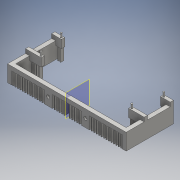
# Autodesk Inventor part: XBOX holder
Saved by Autodesk Inventor 2016 SP2 (Build 200236200, 236)
## iProperties
Created: 2018-02-19
Part Number: XBOX holder
Material: Generic
Document SubType Name: Modeling
Designer: Alexander
Density: 1 g/cm^3
Appearance: Default
Author: Alexander
Autodesk Inventor part; units mm, degrees
ref_plane "YZ Plane" through (0, 0, 0) normal (1, 0, 0) x (0, 1, 0)
ref_plane "XZ Plane" through (0, 0, 0) normal (0, 1, 0) x (-1, 0, 0)
ref_plane "XY Plane" through (0, 0, 0) normal (0, 0, 1) x (1, 0, 0)
sketch "Sketch1" plane through (0, 0, 0) normal (0, 0, 1) x (1, 0, 0)
  line L0 (-57.6, 21) -> (-53.6, 21)
  line L1 (-53.6, 21) -> (-53.6, 17)
  line L2 (-53.6, 17) -> (-57.6, 17)
  line L3 (-57.6, 17) -> (-57.6, 21)
  line L4 (53.6, 21) -> (57.6, 21)
  line L5 (57.6, 21) -> (57.6, 17)
  line L6 (57.6, 17) -> (53.6, 17)
  line L7 (53.6, 17) -> (53.6, 21)
  line L8 (-57.6, 17) -> (-67.6, 17)
  line L9 (-67.6, 17) -> (-67.6, 0)
  line L10 (-67.6, 0) -> (67.6, 0)
  line L11 (67.6, 0) -> (67.6, 17)
  line L12 (67.6, 17) -> (57.6, 17)
  line L13 (-57.6, 21) -> (-53.6, 17) construction
  line L14 (53.6, 17) -> (57.6, 21) construction
  line L15 (-57.6, 21) -> (-72.6, 21)
  line L16 (-72.6, 21) -> (-72.6, -5)
  line L17 (-72.6, -5) -> (72.6, -5)
  line L18 (72.6, -5) -> (72.6, 21)
  line L19 (72.6, 21) -> (57.6, 21)
  point P0 (0, 0)
  point P1 (-55.6, 19)
  point P2 (55.6, 19)
  point P3 (0, 0)
  dimension "d0" = 4
  dimension "d1" = 4
  dimension "d2" = 4
  dimension "d3" = 4
  dimension "d4" = 17
  dimension "d5" = 17
  dimension "d6" = 111.2
  dimension "d7" = 5
  dimension "d8" = 5
  dimension "d9" = 5
  dimension "d10" = 10
  constraints: 40 end point, 7 perpendicular, 5 horizontal, 4 parallel, 3 midpoint, 1 coincident, 1 collinear, 1 point on line, 1 vertical
  measures "d0" distance of L0.start L0.end
  measures "d1" distance of L0.end L1.end
  measures "d2" distance of L4.start L4.end
  measures "d3" distance of L4.end L5.end
  measures "d4" distance of L8.end L9.end
  measures "d5" distance of L10.end L11.end
  measures "d6" distance of point (55.6, 19) point (-55.6, 19)
  measures "d7" distance between parallel lines of L9 L16
  measures "d8" distance between parallel lines of L18 L11
  measures "d9" distance between parallel lines of L17 L10
  measures "d10" distance of L2.end L8.end
extrude "Frame" add sketch "Sketch1" along normal blind 5
sketch "Sketch2" plane through (0, 0, 5) normal (0, 0, 1) x (1, 0, 0)
  line L0 (-67.6, 17) -> (-53.6, 17) projected
  line L1 (-53.6, 17) -> (-57.6, 17)
  line L2 (-57.6, 17) -> (-57.6, 21) construction
  line L3 (-53.6, 21) -> (-72.6, 21) projected
  line L4 (-57.6, 21) -> (-53.6, 17) construction
  circle A0 centre (-55.6, 19) radius 1
  line L5 (0, 0) -> (0, -5.6301) construction
  circle A1 centre (55.6, 19) radius 1
  dimension "d13" = 4
  dimension "d14" = 2
  constraints: 8 end point, 2 centre point, 2 point on line, 1 midpoint, 1 perpendicular, 1 symmetric about line, 1 vertical, 1 other
  measures "d13" distance of L0.end L1.end
  measures "d14" diameter of A0
extrude "Pins" add sketch "Sketch2" along normal blind 10
sketch "Sketch3" plane through (0, 0, 0) normal (0, 0, -1) x (-1, 0, 0)
  line L0 (17.75, -5) -> (-17.75, -5)
  line L1 (72.6, -5) -> (-72.6, -5) projected
  line L2 (72.6, -5) -> (-72.6, -5) projected
  line L3 (17.75, -5) -> (27.75, -5)
  line L4 (27.75, -5) -> (27.75, 0)
  line L5 (27.75, 0) -> (17.75, 0)
  line L6 (17.75, 0) -> (17.75, -5)
  line L7 (0, -5) -> (0, 0) construction
  line L8 (-17.75, -5) -> (-27.75, -5)
  line L9 (-27.75, -5) -> (-27.75, 0)
  line L10 (-27.75, 0) -> (-17.75, 0)
  line L11 (-17.75, 0) -> (-17.75, -5)
  point P0 (0, -5)
  dimension "d17" = 35.5
  dimension "d18" = 10
  dimension "d19" = 5
  constraints: 20 end point, 3 midpoint, 3 symmetric about line, 2 perpendicular, 2 vertical, 1 horizontal, 1 point on line
  measures "d17" distance of L0.start L0.end
  measures "d18" distance of L0.start L3.end
  measures "d19" distance of L3.end L4.end
extrude "Connection Points" add sketch "Sketch3" along normal blind 15
sketch "Sketch4" plane through (-72.6, -5, 5) normal (0, -1, 0) x (1, 0, 0)
  line L0 (44.85, -5) -> (5, -5) projected
  line L1 (44.85, -5) -> (54.85, -5) construction
  line L2 (49.85, -5) -> (49.85, -10) construction
  circle A0 centre (49.85, -10) radius 2
  line L3 (72.6, -5) -> (72.6, 0.0988) construction
  circle A1 centre (95.35, -10) radius 2
  dimension "d22" = 5
  dimension "d23" = 4
  constraints: 6 end point, 2 centre point, 2 vertical, 1 coincident, 1 horizontal, 1 midpoint, 1 symmetric about line, 1 other
  measures "d22" distance of L2.start L2.end
  measures "d23" diameter of A0
extrude "Nail Holes" cut sketch "Sketch4" against normal up to next
sketch "Sketch6" plane through (0, 0, 0) normal (0, 0, -1) x (-1, 0, 0)
  line L0 (-53.6, 17) -> (-67.6, 17) projected
  line L1 (-72.6, 21) -> (-53.6, 21) projected
  line L2 (-67.6, 21) -> (-67.6, 17)
  line L3 (-67.6, 17) -> (-72.6, 17)
  line L4 (-72.6, -5) -> (-72.6, 21) projected
  line L5 (0, 0) -> (0, -5) construction
  line L6 (72.6, -5) -> (-72.6, -5) projected
  line L7 (67.6, 21) -> (67.6, 17)
  line L8 (67.6, 17) -> (72.6, 17)
  line L9 (-72.6, 8) -> (-69.6, 8) construction
  line L10 (-67.6, -5) -> (-67.6, -1)
  line L11 (-67.6, -1) -> (-72.6, -1)
  line L12 (67.6, -1) -> (72.6, -1)
  line L13 (67.6, -5) -> (67.6, -1)
  line L14 (72.6, 21) -> (72.6, -5) projected
  line L15 (53.6, 21) -> (72.6, 21) projected
  line L16 (67.6, -5) -> (72.6, -5)
  line L17 (72.6, -1) -> (72.6, -5)
  line L18 (-72.6, -1) -> (-72.6, -5)
  line L19 (-72.6, -5) -> (-67.6, -5)
  line L20 (67.6, 21) -> (72.6, 21)
  line L21 (72.6, 21) -> (72.6, 17)
  point P0 (72.6, 8)
  point P1 (63.1, 21)
  constraints: 32 end point, 9 symmetric about line, 4 horizontal, 4 midpoint, 3 vertical, 2 point on line, 1 collinear, 1 perpendicular
extrude "Legs" add sketch "Sketch6" along normal blind 15
sketch "Sketch8" plane through (-72.6, 17, 0) normal (0, -1, 0) x (1, 0, 0)
  line L0 (5, 0) -> (5, -15) projected
  line L1 (5, 0) -> (0, 0)
  line L2 (0, -15) -> (0, 5) projected
  line L3 (0, 0) -> (0, -15)
  line L4 (0, -15) -> (5, -15)
  point P0 (72.6, 0)
  constraints: 6 end point, 2 perpendicular, 1 horizontal
extrude "Lower Rim 1" add sketch "Sketch8" along normal up to next
ref_plane "Midplane vertical" through (0, 0, 5) normal (-1, 0, 0) x (0, 0, 1)
mirror "Lower Rim Mirror 1" about plane through (0, 0, 5) normal (-1, 0, 0) of "Lower Rim 1"
sketch "Sketch11" plane through (0, 0, 0) normal (0, 0, -1) x (-1, 0, 0)
  line L0 (-67.6, 21) -> (-53.6, 21)
  line L1 (-53.6, 17) -> (-67.6, 17)
  line L2 (-65.6, 21) -> (-64.6, 21)
  line L3 (-64.6, 21) -> (-64.6, 17)
  line L4 (-64.6, 17) -> (-65.6, 17)
  line L5 (-65.6, 17) -> (-65.6, 21)
  line L6 (-67.6, 17) -> (-67.6, 21)
  line L7 (-62.6, 21) -> (-61.6, 21)
  line L8 (-61.6, 21) -> (-61.6, 17)
  line L9 (-61.6, 17) -> (-62.6, 17)
  line L10 (-62.6, 17) -> (-62.6, 21)
  line L11 (-53.6, 17) -> (-67.6, 17)
  line L12 (-59.6, 21) -> (-58.6, 21)
  line L13 (-58.6, 21) -> (-58.6, 17)
  line L14 (-58.6, 17) -> (-59.6, 17)
  line L15 (-59.6, 17) -> (-59.6, 21)
  line L16 (-56.6, 17) -> (-56.6, 21)
  line L17 (-56.6, 21) -> (-55.6, 21)
  line L18 (-55.6, 17) -> (-56.6, 17)
  line L19 (-55.6, 21) -> (-55.6, 17)
  line L20 (0, 0) -> (0, -5) construction
  line L21 (17.75, -5) -> (-17.75, -5)
  line L22 (53.6, 17) -> (67.6, 17)
  line L23 (53.6, 17) -> (67.6, 17)
  line L24 (67.6, 21) -> (53.6, 21)
  line L25 (59.6, 17) -> (59.6, 21)
  line L26 (59.6, 21) -> (58.6, 21)
  line L27 (58.6, 17) -> (59.6, 17)
  line L28 (58.6, 21) -> (58.6, 17)
  line L29 (56.6, 17) -> (56.6, 21)
  line L30 (55.6, 21) -> (55.6, 17)
  line L31 (55.6, 17) -> (56.6, 17)
  line L32 (56.6, 21) -> (55.6, 21)
  line L33 (65.6, 21) -> (64.6, 21)
  line L34 (64.6, 21) -> (64.6, 17)
  line L35 (62.6, 21) -> (61.6, 21)
  line L36 (61.6, 17) -> (62.6, 17)
  line L37 (61.6, 21) -> (61.6, 17)
  line L38 (64.6, 17) -> (65.6, 17)
  line L39 (65.6, 17) -> (65.6, 21)
  line L40 (67.6, 17) -> (67.6, 21)
  line L41 (62.6, 17) -> (62.6, 21)
  line L42 (-67.6, -5) -> (-67.6, 21) projected
  line L43 (67.6, 21) -> (67.6, -5) projected
  line L44 (64.6, 21) -> (65.6, 21)
  line L45 (65.6, 17) -> (64.6, 17)
  line L46 (67.6, 17) -> (53.6, 17) projected
  point P0 (-62.1, 21)
  point P1 (-62.1, 17)
  point P2 (-59.1, 17)
  point P3 (-59.1, 21)
  point P4 (-56.1, 17)
  point P5 (-56.1, 21)
  point P6 (59.1, 17)
  point P7 (59.1, 21)
  point P8 (56.1, 17)
  point P9 (56.1, 21)
  point P10 (62.1, 21)
  point P11 (62.1, 17)
  point P12 (-67.6, 0)
  point P13 (-67.6, 19)
  point P14 (67.6, 0)
  dimension "d47" = 1
  dimension "d48" = 2
  dimension "d49" = 1
  dimension "d50" = 2
  dimension "d51" = 1
  dimension "d52" = 2
  dimension "d53" = 1
  dimension "d54" = 2
  dimension "d55" = 4
  constraints: 88 end point, 26 symmetric about line, 18 point on line, 8 midpoint, 8 parallel, 4 horizontal, 4 perpendicular, 2 collinear
  measures "d47" distance between parallel lines of L3 L5
  measures "d48" distance between parallel lines of L5 L6
  measures "d49" distance between parallel lines of L8 L10
  measures "d50" distance between parallel lines of L3 L10
  measures "d51" distance between parallel lines of L13 L15
  measures "d52" distance between parallel lines of L15 L8
  measures "d53" distance between parallel lines of L19 L16
  measures "d54" distance between parallel lines of L16 L13
  measures "d55" distance between parallel lines of L1 L0
extrude "Supports Peg" add sketch "Sketch11" along normal blind 15 contours L0 L3 L1 L5 | L0 L8 L1 L10 | L0 L13 L1 L15 | L0 L19 L1 L16 | L30 L24 L29 L22 | L28 L24 L25 L22 | L37 L24 L41 L22 | L34 L24 L39 L22
sketch "Sketch12" plane through (-67.6, 0, 5) normal (0, 1, 0) x (1, 0, 0)
  circle A0 centre (90.35, 10) radius 2 projected
  circle A1 centre (90.35, 10) radius 3
  circle A2 centre (44.85, 10) radius 2 projected
  circle A3 centre (44.85, 10) radius 3
  point P0 (67.6, 5)
  dimension "d58" = 6
  dimension "d59" = 6
  constraints: 2 centre point, 2 coincident
  measures "d58" diameter of A1
  measures "d59" diameter of A3
extrude "Nail Heads" cut sketch "Sketch12" against normal blind 3
sketch "Sketch13" plane through (0, 0, 0) normal (0, 0, -1) x (-1, 0, 0)
  line L0 (27.75, 0) -> (67.6, 0) projected
  line L1 (27.75, 0) -> (29.75, 0)
  line L2 (29.75, 0) -> (29.75, -5)
  line L3 (67.6, -5) -> (27.75, -5) projected
  line L4 (29.75, -5) -> (30.75, -5)
  line L5 (30.75, -5) -> (30.75, 0)
  line L6 (29.75, 0) -> (32.75, 0)
  line L7 (32.75, 0) -> (32.75, -5)
  line L8 (32.75, -5) -> (33.75, -5)
  line L9 (33.75, -5) -> (33.75, 0)
  line L10 (32.75, 0) -> (33.75, 0)
  line L11 (33.75, 0) -> (35.75, 0)
  line L12 (35.75, 0) -> (35.75, -5)
  line L13 (35.75, -5) -> (36.75, -5)
  line L14 (36.75, -5) -> (36.75, 0)
  line L15 (35.75, 0) -> (36.75, 0)
  line L16 (36.75, 0) -> (38.75, 0)
  line L17 (38.75, 0) -> (38.75, -5)
  line L18 (38.75, -5) -> (39.75, -5)
  line L19 (39.75, -5) -> (39.75, 0)
  line L20 (38.75, 0) -> (39.75, 0)
  line L21 (39.75, 0) -> (41.75, 0)
  line L22 (41.75, 0) -> (41.75, -5)
  line L23 (41.75, -5) -> (42.75, -5)
  line L24 (42.75, -5) -> (42.75, 0)
  line L25 (41.75, 0) -> (42.75, 0)
  line L26 (42.75, 0) -> (44.75, 0)
  line L27 (44.75, 0) -> (44.75, -5)
  line L28 (44.75, -5) -> (45.75, -5)
  line L29 (45.75, -5) -> (45.75, 0)
  line L30 (44.75, 0) -> (45.75, 0)
  line L31 (45.75, 0) -> (47.75, 0)
  line L32 (47.75, 0) -> (47.75, -5)
  line L33 (72.6, -5) -> (-72.6, -5) projected
  line L34 (47.75, -5) -> (48.75, -5)
  line L35 (48.75, -5) -> (48.75, 0)
  line L36 (-67.6, 0) -> (67.6, 0) projected
  line L37 (47.8501, 0) -> (48.75, 0)
  line L38 (48.75, 0) -> (50.75, 0)
  line L39 (50.75, 0) -> (50.75, -5)
  line L40 (50.75, -5) -> (51.75, -5)
  line L41 (51.75, -5) -> (51.75, 0)
  line L42 (50.75, 0) -> (51.75, 0)
  line L43 (51.75, 0) -> (50.75, 0)
  line L44 (51.75, 0) -> (53.75, 0)
  line L45 (53.75, 0) -> (53.75, -5)
  line L46 (53.75, -5) -> (54.75, -5)
  line L47 (54.75, -5) -> (54.75, 0)
  line L48 (53.75, 0) -> (54.75, 0)
  line L49 (54.75, 0) -> (56.75, 0)
  line L50 (56.75, 0) -> (56.75, -5)
  line L51 (56.75, -5) -> (57.75, -5)
  line L52 (57.75, -5) -> (57.75, 0)
  line L53 (56.75, 0) -> (57.75, 0)
  line L54 (57.75, 0) -> (59.75, 0)
  line L55 (59.75, 0) -> (59.75, -5)
  line L56 (59.75, -5) -> (60.75, -5)
  line L57 (60.75, -5) -> (60.75, 0)
  line L58 (59.75, 0) -> (60.75, 0)
  line L59 (60.75, 0) -> (62.75, 0)
  line L60 (62.75, 0) -> (62.75, -5)
  line L61 (62.75, -5) -> (63.75, -5)
  line L62 (63.75, -5) -> (63.75, 0)
  line L63 (62.75, 0) -> (63.75, 0)
  line L64 (63.75, 0) -> (65.75, 0)
  line L65 (65.75, 0) -> (65.75, -5)
  line L66 (65.75, -5) -> (66.75, -5)
  line L67 (66.75, -5) -> (66.75, 0)
  line L68 (65.75, 0) -> (66.75, 0)
  line L69 (47.8501, 0) -> (47.75, 0)
  point P0 (0, 0)
  dimension "d62" = 2
  dimension "d63" = 1
  dimension "d64" = 3
  dimension "d65" = 1
  dimension "d66" = 2
  dimension "d67" = 1
  dimension "d68" = 2
  dimension "d69" = 1
  dimension "d70" = 2
  dimension "d71" = 1
  dimension "d72" = 2
  dimension "d73" = 1
  dimension "d74" = 2
  dimension "d75" = 1
  dimension "d76" = 2
  dimension "d77" = 1
  dimension "d78" = 2
  dimension "d79" = 1
  dimension "d80" = 2
  dimension "d81" = 1
  dimension "d82" = 2
  dimension "d83" = 1
  dimension "d84" = 2
  dimension "d85" = 1
  dimension "d86" = 2
  dimension "d87" = 1
  constraints: 132 end point, 25 vertical, 8 perpendicular, 7 horizontal, 57 other
  measures "d62" distance of L1.start L1.end
  measures "d63" distance of L2.end L4.end
  measures "d64" distance of L1.end L6.end
  measures "d65" distance of L7.end L8.end
  measures "d66" distance of L9.end L11.end
  measures "d67" distance of L12.end L13.end
  measures "d68" distance of L14.end L16.end
  measures "d69" distance of L17.end L18.end
  measures "d70" distance of L19.end L21.end
  measures "d71" distance of L22.end L23.end
  measures "d72" distance of L24.end L26.end
  measures "d73" distance of L27.end L28.end
  measures "d74" distance of L29.end L31.end
  measures "d75" distance of L32.end L34.end
  measures "d76" distance of L35.end L38.end
  measures "d77" distance of L39.end L40.end
  measures "d78" distance of L41.end L44.end
  measures "d79" distance of L45.end L46.end
  measures "d80" distance of L47.end L49.end
  measures "d81" distance of L50.end L51.end
  measures "d82" distance of L52.end L54.end
  measures "d83" distance of L55.end L56.end
  measures "d84" distance of L57.end L59.end
  measures "d85" distance of L60.end L61.end
  measures "d86" distance of L62.end L64.end
  measures "d87" distance of L65.end L66.end
extrude "Supports Front" add sketch "Sketch13" along normal blind 15 contours L0 L5 L3 L2 | L0 L9 L3 L7 | L0 L14 L3 L12 | L0 L19 L3 L17 | L0 L24 L3 L22 | L0 L29 L3 L27 | L0 L35 L3 L32 | L0 L41 L3 L39 | L0 L47 L3 L45 | L0 L52 L3 L50 | L0 L57 L3 L55 | L0 L62 L3 L60 | L0 L67 L3 L65
mirror "Mirror3" about plane through (0, 0, 5) normal (-1, 0, 0) of "Supports Front"
sketch "Sketch14" plane through (0, 0, 0) normal (0, 0, -1) x (-1, 0, 0)
  line L0 (17.75, -5) -> (-17.75, -5) construction
  line L1 (17.75, -5) -> (15.75, -5)
  line L2 (15.75, -5) -> (15.75, 0)
  line L3 (15.75, 0) -> (14.75, 0)
  line L4 (-17.75, 0) -> (17.75, 0) construction
  line L5 (14.75, 0) -> (14.75, -5)
  line L6 (15.75, -5) -> (14.75, -5)
  line L7 (14.75, 0) -> (12.75, 0)
  line L8 (12.75, 0) -> (12.75, -5)
  line L9 (12.75, -5) -> (11.75, -5)
  line L10 (11.75, -5) -> (11.75, 0)
  line L11 (12.75, 0) -> (11.75, 0)
  line L12 (11.75, -5) -> (9.75, -5)
  line L13 (9.75, -5) -> (9.75, 0)
  line L14 (9.75, 0) -> (8.75, 0)
  line L15 (8.75, 0) -> (8.75, -5)
  line L16 (9.75, -5) -> (8.75, -5)
  line L17 (8.75, -5) -> (6.75, -5)
  line L18 (6.75, -5) -> (6.75, 0)
  line L19 (6.75, 0) -> (5.75, 0)
  line L20 (5.75, 0) -> (5.75, -5)
  line L21 (6.75, -5) -> (5.75, -5)
  line L22 (5.75, -5) -> (3.75, -5)
  line L23 (3.75, -5) -> (3.75, 0)
  line L24 (3.75, -5) -> (2.75, -5)
  line L25 (72.6, -5) -> (-72.6, -5) projected
  line L26 (2.75, -5) -> (2.75, 0)
  line L27 (3.75, 0) -> (2.75, 0)
  line L28 (2.75, -5) -> (0.75, -5)
  point P0 (0, 0)
  dimension "d90" = 2
  dimension "d91" = 1
  dimension "d92" = 5
  dimension "d93" = 2
  dimension "d94" = 1
  dimension "d95" = 2
  dimension "d96" = 1
  dimension "d97" = 2
  dimension "d98" = 1
  dimension "d99" = 2
  dimension "d100" = 1
  dimension "d101" = 2
  constraints: 52 end point, 6 vertical, 5 horizontal, 4 perpendicular, 2 point on line, 20 other
  measures "d90" distance of L1.start L1.end
  measures "d91" distance of L2.end L3.end
  measures "d92" distance of L1.end L2.end
  measures "d93" distance of L3.end L7.end
  measures "d94" distance of L8.end L9.end
  measures "d95" distance of L9.end L12.end
  measures "d96" distance of L13.end L14.end
  measures "d97" distance of L15.end L17.end
  measures "d98" distance of L18.end L19.end
  measures "d99" distance of L20.end L22.end
  measures "d100" distance of L22.end L24.end
  measures "d101" distance of L24.end L28.end
extrude "Internal Supports Front" add sketch "Sketch14" along normal blind 15 contours L6 L5 L3 L2 | L24 L26 L27 L23 | L21 L20 L19 L18 | L16 L15 L14 L13 | L9 L10 L11 L8
mirror "Mirror4" about plane through (0, 0, 5) normal (-1, 0, 0) of "Internal Supports Front"
sketch "Sketch15" plane through (-72.6, 21, 5) normal (0, 1, 0) x (1, 0, 0)
  line L0 (140.2, 5) -> (140.2, 20) projected
  line L1 (140.2, 5) -> (140.2, 0) projected
  line L2 (140.2, 20) -> (140.2, 0)
  line L3 (140.2, 0) -> (145.2, 0)
  line L4 (145.2, 20) -> (145.2, 0) projected
  line L5 (145.2, 0) -> (145.2, 20)
  line L6 (145.2, 20) -> (140.2, 20)
  line L7 (5, 5) -> (5, 0) projected
  line L8 (5, 0) -> (5, 20)
  line L9 (0, 20) -> (5, 20) projected
  line L10 (5, 20) -> (0, 20)
  line L11 (0, 20) -> (0, 0) projected
  line L12 (0, 20) -> (0, 0)
  line L13 (0, 0) -> (5, 0)
  point P0 (72.6, 5)
  constraints: 16 end point, 6 perpendicular, 2 vertical
extrude "Side Frame Extension" add sketch "Sketch15" along normal blind 40
sketch "Sketch16" plane through (67.6, 0, 5) normal (-1, 0, 0) x (0, 0, 1)
  line L0 (0, 21) -> (0, 61) projected
  line L1 (0, 52.928) -> (-5, 52.928)
  line L2 (-5, 52.928) -> (-5, 48.928)
  line L3 (-5, 48.928) -> (0, 48.928)
  line L4 (0, 48.928) -> (0, 52.928)
  line L5 (-5, 17) -> (0, 17) projected
  line L6 (0, 17) -> (0, 21)
  point P0 (-5, 0)
  point P1 (0, 19)
  point P2 (0, 50.928)
  dimension "d106" = 5
  dimension "d107" = 4
  dimension "d108" = 31.928
  constraints: 10 end point, 2 midpoint, 2 parallel, 1 horizontal, 1 perpendicular, 1 point on line, 1 vertical
  measures "d106" distance of L3.end L2.end
  measures "d107" distance of L1.end L2.end
  measures "d108" distance of point (0, 19) point (0, 50.928)
extrude "Back Bar" add sketch "Sketch16" along normal blind 7
mirror "Between two Rows" about plane through (0, 0, 5) normal (-1, 0, 0) of "Back Bar"
sketch "Sketch17" plane through (0, 0, 5) normal (0, 0, 1) x (1, 0, 0)
  circle A0 centre (-55.6, 19) radius 1 projected
  circle A1 centre (-55.6, 19) radius 2
  point P0 (0, 0)
  dimension "d111" = 4
  constraints: 1 centre point, 1 coincident
  measures "d111" diameter of A1
extrude "BoxRest" add sketch "Sketch17" along normal blind 5
mirror "Mirror6" about plane through (0, 0, 5) normal (-1, 0, 0) of "BoxRest"
sketch "Sketch18" plane through (0, 0, 5) normal (0, 0, 1) x (1, 0, 0)
  line L0 (-67.6, 52.928) -> (-60.6, 52.928) projected
  line L1 (-67.6, 48.928) -> (-60.6, 48.928) projected
  line L2 (67.6, 48.928) -> (60.6, 48.928) projected
  circle A0 centre (-62.765, 50.928) radius 2
  circle A1 centre (62.765, 50.928) radius 2
  line L3 (-72.6, -5) -> (-72.6, 61) projected
  line L4 (62.765, 50.928) -> (72.6, 50.928) construction
  line L5 (72.6, -5) -> (72.6, 61) projected
  line L6 (-72.6, 50.928) -> (-62.765, 50.928) construction
  point P0 (0, 0)
  dimension "d114" = 4
  dimension "d115" = 4
  dimension "d116" = 125.53
  constraints: 4 end point, 2 centre point, 2 horizontal, 2 point on line, 1 collinear
  measures "d114" diameter of A0
  measures "d115" diameter of A1
  measures "d116" distance of L4.start L6.end
extrude "Front peg bottoms" add sketch "Sketch18" along normal blind 5
sketch "Sketch19" plane through (-62.765, 50.928, 10) normal (0, 0, 1) x (1, 0, 0)
  circle A0 centre (0, 0) radius 1
  point P0 (62.765, -50.928)
  dimension "d119" = 2
  constraints: 1 centre point
  measures "d119" diameter of A0
extrude "Front peg tops" add sketch "Sketch19" along normal blind 5
mirror "Mirror7" about plane through (0, 0, 5) normal (-1, 0, 0) of "Front peg tops"
sketch "Sketch20" plane through (67.6, 48.928, 0) normal (0, 0, -1) x (-1, 0, 0)
  line L0 (2, 4) -> (3, 4)
  line L1 (3, 4) -> (3, 0)
  line L2 (3, 0) -> (2, 0)
  line L3 (2, 0) -> (2, 4)
  line L4 (0, 4) -> (7, 4) construction
  line L5 (0, 0) -> (7, 0) construction
  line L6 (0, -27.928) -> (0, 0) projected
  line L7 (0, 0) -> (7, 0)
  line L8 (0, 4) -> (7, 4)
  line L9 (0, 4) -> (0, 0) construction
  line L10 (0, -53.928) -> (0, 12.072) projected
  line L11 (5, 4) -> (6, 4)
  line L12 (6, 4) -> (6, 0)
  line L13 (6, 0) -> (5, 0)
  line L14 (5, 0) -> (5, 4)
  point P0 (67.6, -48.928)
  point P1 (3.5, 0)
  point P2 (2.5, 4)
  point P3 (5.5, 4)
  point P4 (5.5, 0)
  dimension "d122" = 4
  dimension "d123" = 2
  dimension "d124" = 1
  dimension "d125" = 2
  dimension "d126" = 1
  constraints: 22 end point, 4 midpoint, 4 parallel, 3 collinear, 3 point on line, 2 horizontal, 2 perpendicular
  measures "d122" distance of L0.end L1.end
  measures "d123" distance between parallel lines of L9 L3
  measures "d124" distance between parallel lines of L1 L3
  measures "d125" distance between parallel lines of L14 L1
  measures "d126" distance between parallel lines of L12 L14
extrude "Front Supports" add sketch "Sketch20" along normal blind 15 contours L0 L1 L2 L3 | L8 L12 L7 L14
mirror "Mirror8" about plane through (0, 0, 5) normal (-1, 0, 0) of "Front Supports"
sketch "Sketch21" plane through (-72.6, 61, 5) normal (0, 1, 0) x (1, 0, 0)
  line L0 (0, 0) -> (145.2, 0) projected
  line L1 (140.2, 0) -> (145.2, 0)
  line L2 (145.2, 20) -> (145.2, 0) projected
  line L3 (145.2, 0) -> (145.2, 20)
  line L4 (145.2, 20) -> (140.2, 20)
  line L5 (140.2, 20) -> (140.2, 0)
  line L6 (140.2, 20) -> (140.2, 0) projected
  line L7 (0, 20) -> (0, 0) projected
  line L8 (0, 0) -> (0, 20)
  line L9 (0, 20) -> (5, 20)
  line L10 (5, 20) -> (5, 0)
  line L11 (5, 0) -> (5, 20) projected
  point P0 (72.6, 5)
  point P1 (140.2, 10)
  point P2 (140.2, 10)
  point P3 (5, 10)
  point P4 (5, 10)
  constraints: 14 end point, 6 midpoint, 5 perpendicular, 2 point on line, 1 collinear, 1 horizontal
extrude "Resizing" cut sketch "Sketch21" against normal blind 8.072
sketch "Sketch22" plane through (0, 0, 5) normal (0, 0, 1) x (1, 0, 0)
  line L0 (-72.6, -5) -> (-72.6, 52.928) projected
  line L1 (-60.6, 52.928) -> (-72.6, 52.928)
  line L2 (-72.6, 52.928) -> (-72.6, 48.928)
  line L3 (-72.6, 48.928) -> (-60.6, 48.928)
  line L4 (-60.6, 48.928) -> (-60.6, 52.928)
  line L5 (-60.6, 48.928) -> (-60.6, 52.928) projected
  line L6 (-67.6, -5) -> (-67.6, 52.928) construction
  line L7 (-67.6, 48.928) -> (-67.6, 21)
  line L8 (0, 0) -> (0, -5) construction
  line L9 (-53.6, 17) -> (-53.6, 21) projected
  line L10 (-53.6, 21) -> (-72.6, 21)
  line L11 (-72.6, 21) -> (-72.6, 17)
  line L12 (-72.6, 17) -> (-53.6, 17)
  line L13 (-53.6, 17) -> (-53.6, 21)
  line L14 (-67.6, 17) -> (-55.6, 17) projected
  line L15 (60.6, 52.928) -> (72.6, 52.928)
  line L16 (72.6, 52.928) -> (72.6, 48.928)
  line L17 (72.6, 48.928) -> (60.6, 48.928)
  line L18 (60.6, 48.928) -> (60.6, 52.928)
  line L19 (60.6, 48.928) -> (60.6, 52.928)
  line L20 (67.6, 48.928) -> (67.6, 21)
  line L21 (53.6, 17) -> (53.6, 21)
  line L22 (53.6, 21) -> (72.6, 21)
  line L23 (72.6, 21) -> (72.6, 17)
  line L24 (72.6, 17) -> (53.6, 17)
  line L25 (53.6, 17) -> (53.6, 21)
  line L26 (67.6, 17) -> (55.6, 17)
  point P0 (-60.6, 50.928)
  point P1 (-62.765, 52.928)
  point P2 (-62.765, 48.928)
  point P3 (-61.6, 17)
  point P4 (72.6, 52.928)
  point P5 (60.6, 50.928)
  point P6 (62.765, 52.928)
  point P7 (62.765, 48.928)
  point P8 (67.6, 52.928)
  point P9 (61.6, 17)
  constraints: 44 end point, 21 symmetric about line, 11 point on line, 4 midpoint, 4 parallel, 2 horizontal, 2 perpendicular, 1 collinear, 1 vertical
extrude "Robust peg bottoms" add sketch "Sketch22" along normal blind 5 contours L0 L10 L9 L12 | L0 L1 L4 L3 | L22 L23 L24 L21 | L15 L16 L17 L18
body "Solid1"
